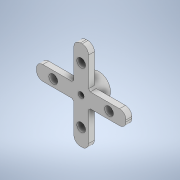
# Autodesk Inventor part: ServoESP32Arm
Saved by Autodesk Inventor 2020 (Build 240168000, 168)
## iProperties
Created: 2022-11-25
Part Number: ServoESP32Arm
Material: Generic
Document SubType Name: Modeling
Designer: agraa4529
Density: 1 g/cm^3
Appearance: Default
Author: agraa4529
Autodesk Inventor part; units mm, degrees
ref_plane "YZ Plane" through (0, 0, 0) normal (1, 0, 0) x (0, 1, 0)
ref_plane "XZ Plane" through (0, 0, 0) normal (0, 1, 0) x (-1, 0, 0)
ref_plane "XY Plane" through (0, 0, 0) normal (0, 0, 1) x (1, 0, 0)
sketch "Sketch2" plane through (0, 0, 0) normal (0, 0, 1) x (1, 0, 0)
  circle A0 centre (0, 0) radius 4
  line L0 (0, 2.05) -> (0, 2.75)
  line L1 (0, 2.75) -> (-0.3545, 2.0191)
  line L2 (0, 2.75) -> (0.3545, 2.0191)
  line L3 (-0.9406, 2.5842) -> (-1.0237, 1.7761)
  line L4 (-0.9406, 2.5842) -> (-0.3574, 2.0186)
  line L5 (-1.7677, 2.1066) -> (-1.5694, 1.3189)
  line L6 (-1.7677, 2.1066) -> (-1.0263, 1.7746)
  line L7 (-2.3816, 1.375) -> (-1.9259, 0.7025)
  line L8 (-2.3816, 1.375) -> (-1.5713, 1.3166)
  line L9 (-2.7082, 0.4775) -> (-2.05, 0.0015)
  line L10 (-2.7082, 0.4775) -> (-1.9269, 0.6997)
  line L11 (-2.7082, -0.4775) -> (-1.9269, -0.6997)
  line L12 (-2.7082, -0.4775) -> (-2.05, -0.0015)
  line L13 (-2.3816, -1.375) -> (-1.5713, -1.3166)
  line L14 (-2.3816, -1.375) -> (-1.9259, -0.7025)
  line L15 (-1.7677, -2.1066) -> (-1.0263, -1.7746)
  line L16 (-1.7677, -2.1066) -> (-1.5694, -1.3189)
  line L17 (-0.9406, -2.5842) -> (-0.3574, -2.0186)
  line L18 (-0.9406, -2.5842) -> (-1.0237, -1.7761)
  line L19 (0, -2.75) -> (0.3545, -2.0191)
  line L20 (0, -2.75) -> (-0.3545, -2.0191)
  line L21 (0.9406, -2.5842) -> (1.0237, -1.7761)
  line L22 (0.9406, -2.5842) -> (0.3574, -2.0186)
  line L23 (1.7677, -2.1066) -> (1.5694, -1.3189)
  line L24 (1.7677, -2.1066) -> (1.0263, -1.7746)
  line L25 (2.3816, -1.375) -> (1.9259, -0.7025)
  line L26 (2.3816, -1.375) -> (1.5713, -1.3166)
  line L27 (2.7082, -0.4775) -> (2.05, -0.0015)
  line L28 (2.7082, -0.4775) -> (1.9269, -0.6997)
  line L29 (2.7082, 0.4775) -> (1.9269, 0.6997)
  line L30 (2.7082, 0.4775) -> (2.05, 0.0015)
  line L31 (2.3816, 1.375) -> (1.5713, 1.3166)
  line L32 (2.3816, 1.375) -> (1.9259, 0.7025)
  line L33 (1.7677, 2.1066) -> (1.0263, 1.7746)
  line L34 (1.7677, 2.1066) -> (1.5694, 1.3189)
  line L35 (0.9406, 2.5842) -> (0.3574, 2.0186)
  line L36 (0.9406, 2.5842) -> (1.0237, 1.7761)
  arc A1 (-1.9259, 0.7025) -> (-1.9269, 0.6997) centre (0, 0) ccw
  arc A2 (-2.05, 0.0015) -> (-2.05, -0.0015) centre (0, 0) ccw
  arc A3 (-1.9269, -0.6997) -> (-1.9259, -0.7025) centre (0, 0) ccw
  arc A4 (-1.5713, -1.3166) -> (-1.5694, -1.3189) centre (0, 0) ccw
  arc A5 (-1.0263, -1.7746) -> (-1.0237, -1.7761) centre (0, 0) ccw
  arc A6 (-0.3574, -2.0186) -> (-0.3545, -2.0191) centre (0, 0) ccw
  arc A7 (0.3545, -2.0191) -> (0.3574, -2.0186) centre (0, 0) ccw
  arc A8 (1.0237, -1.7761) -> (1.0263, -1.7746) centre (0, 0) ccw
  arc A9 (1.5694, -1.3189) -> (1.5713, -1.3166) centre (0, 0) ccw
  arc A10 (1.9259, -0.7025) -> (1.9269, -0.6997) centre (0, 0) ccw
  arc A11 (2.05, -0.0015) -> (2.05, 0.0015) centre (0, 0) ccw
  arc A12 (1.9269, 0.6997) -> (1.9259, 0.7025) centre (0, 0) ccw
  arc A13 (1.5713, 1.3166) -> (1.5694, 1.3189) centre (0, 0) ccw
  arc A14 (1.0263, 1.7746) -> (1.0237, 1.7761) centre (0, 0) ccw
  arc A15 (0.3574, 2.0186) -> (0.3545, 2.0191) centre (0, 0) ccw
  arc A16 (-0.3545, 2.0191) -> (-0.3574, 2.0186) centre (0, 0) ccw
  arc A17 (-1.0237, 1.7761) -> (-1.0263, 1.7746) centre (0, 0) ccw
  arc A18 (-1.5694, 1.3189) -> (-1.5713, 1.3166) centre (0, 0) ccw
  dimension "d7" = 8
  dimension "d9" = 0.7
  dimension "d12" = 360
  constraints: 74 end point, 36 point on circle, 19 centre point, 2 coincident, 1 vertical, 91 other
  measures "d7" diameter of A0
  measures "d9" distance of L0.start L0.end
extrude "Extrusion1" add sketch "Sketch2" along normal blind 4
sketch "Sketch3" plane through (0, 0, 4) normal (0, 0, 1) x (1, 0, 0)
  circle A0 centre (0, 0) radius 1
  circle A1 centre (0, 0) radius 4
  dimension "d16" = 2
  constraints: 2 centre point, 2 coincident
  measures "d16" diameter of A0
extrude "Extrusion2" add sketch "Sketch3" along normal blind 2
sketch "Sketch4" plane through (0, 0, 6) normal (0, 0, 1) x (1, 0, 0)
  circle A0 centre (0, 0) radius 4 projected
  line L0 (-2.5, 15.2615) -> (2.5, 15.2615)
  line L1 (2.5, 15.2615) -> (2.5, 3.7385)
  line L2 (-2.5, 3.7385) -> (-2.5, 15.2615)
  line L3 (-2.5, 15.2615) -> (2.5, 3.7385) construction
  line L4 (2.5, 15.2615) -> (-2.5, 3.7385) construction
  line L5 (2.5, 3.7385) -> (2.5, 3.1225)
  line L6 (2.5, 3.1225) -> (-2.5, 3.1225)
  line L7 (-2.5, 3.1225) -> (-2.5, 3.7385)
  line L8 (-3.7385, -2.5) -> (-15.2615, -2.5)
  line L9 (-15.2615, -2.5) -> (-15.2615, 2.5)
  line L10 (-15.2615, 2.5) -> (-3.7385, 2.5)
  line L11 (-3.1225, 2.5) -> (-3.1225, -2.5)
  line L12 (-3.1225, -2.5) -> (-3.7385, -2.5)
  line L13 (-3.7385, 2.5) -> (-3.1225, 2.5)
  line L14 (2.5, -3.7385) -> (2.5, -15.2615)
  line L15 (2.5, -15.2615) -> (-2.5, -15.2615)
  line L16 (-2.5, -15.2615) -> (-2.5, -3.7385)
  line L17 (-2.5, -3.1225) -> (2.5, -3.1225)
  line L18 (2.5, -3.1225) -> (2.5, -3.7385)
  line L19 (-2.5, -3.7385) -> (-2.5, -3.1225)
  line L20 (3.7385, 2.5) -> (15.2615, 2.5)
  line L21 (15.2615, 2.5) -> (15.2615, -2.5)
  line L22 (15.2615, -2.5) -> (3.7385, -2.5)
  line L23 (3.1225, -2.5) -> (3.1225, 2.5)
  line L24 (3.1225, 2.5) -> (3.7385, 2.5)
  line L25 (3.7385, -2.5) -> (3.1225, -2.5)
  circle A1 centre (9.5, 0) radius 1.5
  circle A2 centre (0, 9.5) radius 1.5
  circle A3 centre (-9.5, 0) radius 1.5
  circle A4 centre (0, -9.5) radius 1.5
  point P0 (0, 9.5)
  point P1 (-3.1225, -2.5)
  dimension "d20" = 5
  dimension "d21" = 11.523
  dimension "d22" = 0.616
  dimension "d23" = 5
  dimension "d26" = 360
  dimension "d31" = 3
  dimension "d34" = 360
  constraints: 52 end point, 4 centre point, 2 midpoint, 2 parallel, 1 horizontal, 1 perpendicular, 64 other
  measures "d20" distance of L1.end L2.start
  measures "d21" distance of L0.end L1.end
  measures "d22" distance of L5.start L5.end
  measures "d23" distance of L0.start L0.end
  measures "d31" diameter of A1
extrude "Extrusion3" add sketch "Sketch4" against normal blind 2 contours A0 L24 L20 L21 L22 L25 | A0 L7 L2 L0 L1 L5 | L18 L14 L15 L16 L19 A0 | A0 L12 L8 L9 L10 L13
fillet "Fillet1" radius 2.2 8 edges at (2.5, -15.2615, 5) (-15.2615, -2.5, 5) (-15.2615, 2.5, 5) (-2.5, 15.2615, 5) (2.5, 15.2615, 5) (15.2615, 2.5, 5) (15.2615, -2.5, 5) (-2.5, -15.2615, 5)
body "Solid1"
